Autodesk Fusion 360 part; units mm, degrees
(part 2 of 2)
equation "magOD = 6.2 mm" comment "5.88 mm"
equation "buttonOD = 28 mm"
equation "buttonH = 9.9 mm"
equation "baseMagW = 48 mm"
equation "coverMagH = 15 mm"
equation "screwHoleDFC = 21 mm"
equation "d178 = 28.40 mm"
equation "NeopixelCoverSupportOD = 26.4 mm"
equation "screwHeadheight = 1.2954 mm"
equation "baseLipH = 3.175 mm"
equation "capBaseW = 39 mm"
equation "capBaseL = 39 mm"
equation "d43 = capsenseWidth"
equation "d44 = capsenseLength"
equation "d45 = ( 34 / 2 ) * 1 mm"
equation "d46 = capsenseWidth / 2"
equation "d50 = magOD"
equation "d58 = capsenseLength / 2"
equation "d59 = capsenseWidth / 2"
equation "magnetDepth = -1.7 mm" comment "1.43 mm"
equation "d61 = magnetDepth"
equation "d64 = capsenseThick + 0.2 mm"
equation "d67 = capsenseWidth"
equation "d69 = ( 34 / 2 ) * 1 mm"
equation "d70 = capsenseWidth / 2"
equation "d86 = capBaseW"
equation "d87 = capBaseL"
equation "d90 = buttonOD"
equation "d91 = buttonH + 3 mm"
equation "magCentertoCapsense = 4.2 mm"
equation "d106 = magnetDepth"
equation "d108 = magnetDepth"
equation "d114 = capBaseW / 2"
equation "d115 = capBaseW / 2"
equation "d116 = screwHoleID"
equation "d123 = screwHole_OD"
equation "d125 = -screwHeadheight"
equation "d140 = buttonOD + 1 mm"
equation "d149 = boxW"
equation "boxW = 70 mm"
equation "boxH = 50 mm"
equation "boxTopH = 3 mm"
equation "d196 = screwHoleID"
equation "d197 = screwHoleID"
equation "d216 = boxW / 2"
equation "boxL = 100 mm"
equation "d249 = ( 65.8 / 2 ) * 1 mm"
equation "d250 = ( 95.8 / 2 ) * 1 mm"
equation "d253 = buttonOD + 0.5 mm"
equation "d254 = ( 39 / 2 ) * 1 mm"
equation "d256 = ( 39 / 2 ) * 1 mm"
equation "d257 = ( 39 / 2 ) * 1 mm"
equation "d353 = 55 mm - 3.175 mm - 0.2 mm + 3 mm"
equation "d359 = ( 95.5 / 2 ) * 1 mm"
equation "d360 = ( 35 / 2 ) * 1 mm"
equation "d365 = ( 39 / 2 ) * 1 mm"
equation "d367 = ( 39 / 2 ) * 1 mm"
equation "d368 = capsenseWidth"
equation "d369 = capsenseLength"
equation "d370 = capsenseLength / 2"
equation "d371 = capsenseWidth / 2"
equation "d372 = magOD"
